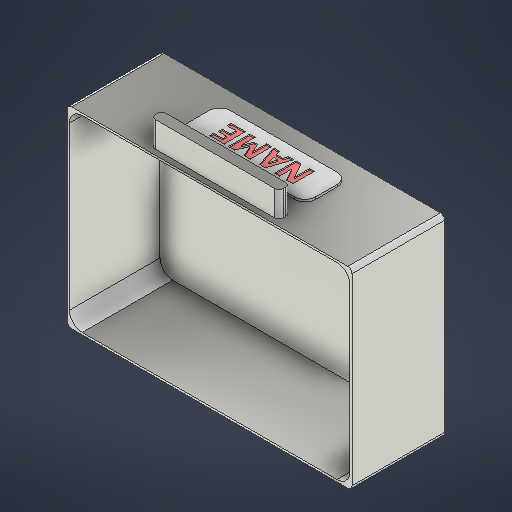
# Autodesk Inventor part: shelf1x2
Saved by Autodesk Inventor 2027 (Build 310192060, 192F)
## iProperties
Created: 2026-06-08
Part Number: shelf1x2
Material: Ogólny
Document SubType Name: Modeling
Designer: User
Density: 1 g/cm^3
Appearance: Domyślna
Author: User
Autodesk Inventor part; units mm, degrees
ref_plane "YZ Plane" through (0, 0, 0) normal (1, 0, 0) x (0, 1, 0)
ref_plane "XZ Plane" through (0, 0, 0) normal (0, 1, 0) x (-1, 0, 0)
ref_plane "XY Plane" through (0, 0, 0) normal (0, 0, 1) x (1, 0, 0)
sketch "Szkic1" plane through (0, 0, 0) normal (0, 1, 0) x (-1, 0, 0)
  line L0 (-66.7, -21.7) -> (66.7, -21.7)
  line L1 (66.7, -21.7) -> (66.7, 21.7)
  line L2 (66.7, 21.7) -> (-66.7, 21.7)
  line L3 (-66.7, 21.7) -> (-66.7, -21.7)
  line L4 (-66.7, -21.7) -> (66.7, 21.7) construction
  line L5 (66.7, -21.7) -> (-66.7, 21.7) construction
  point P0 (0, 0)
  dimension "d0" = 133.4
  dimension "d1" = 43.4
  constraints: 12 end point, 2 midpoint, 2 parallel, 1 horizontal, 1 perpendicular
  measures "d0" distance of L2.end L1.end
  measures "d1" distance of L1.end L0.end
extrude "Wyciągnięcie proste1" add sketch "Szkic1" along normal blind 90
shell "Skorupa1" thickness 1 removed faces 1 at (-22.2333, 30, 21.7)
sketch "Szkic2" plane through (0, 90, 0) normal (0, 1, 0) x (1, 0, 0)
  line L0 (-66.7, -21.7) -> (66.7, -21.7) projected
  line L1 (0, -21.7) -> (0, -16.7)
  line L2 (30, -19.2) -> (-30, -19.2)
  line L3 (-30, -19.2) -> (-30, -14.2)
  line L4 (-30, -14.2) -> (30, -14.2)
  line L5 (30, -14.2) -> (30, -19.2)
  line L6 (30, -19.2) -> (-30, -14.2) construction
  line L7 (-30, -19.2) -> (30, -14.2) construction
  point P0 (0, 0)
  dimension "d5" = 5
  dimension "d6" = 60
  dimension "d7" = 5
  constraints: 14 end point, 3 midpoint, 2 parallel, 1 horizontal, 1 perpendicular, 1 vertical
  measures "d5" distance of L1.start L1.end
  measures "d6" distance of L2.start L2.end
  measures "d7" distance of L2.end L3.end
extrude "Wyciągnięcie proste2" add sketch "Szkic2" along normal blind 12
sketch "Szkic3" plane through (0, 90, 0) normal (0, 1, 0) x (1, 0, 0)
  line L0 (0, 0) -> (0, 3)
  line L1 (30, 13) -> (-30, 13)
  line L2 (-30, 13) -> (-30, -7)
  line L3 (-30, -7) -> (30, -7)
  line L4 (30, -7) -> (30, 13)
  line L5 (30, 13) -> (-30, -7) construction
  line L6 (-30, 13) -> (30, -7) construction
  dimension "d10" = 3
  dimension "d11" = 60
  dimension "d12" = 20
  constraints: 14 end point, 2 midpoint, 2 parallel, 1 horizontal, 1 perpendicular, 1 vertical
  measures "d10" distance of L0.start L0.end
  measures "d11" distance of L3.end L2.end
  measures "d12" distance of L2.end L1.end
extrude "Wyciągnięcie proste3" add sketch "Szkic3" along normal blind 1
sketch "Szkic4" plane through (0, 91, 0) normal (0, 1, 0) x (1, 0, 0)
  line L0 (30, -7) -> (-30, -7) construction
  line L1 (-30, -7) -> (-30, 13) construction
  line L2 (-30, 13) -> (30, 13) construction
  line L3 (30, 13) -> (30, -7) construction
  line L4 (-30, -7) -> (30, -7) projected
  line L5 (-30, 13) -> (-30, -7) projected
  line L6 (30, -7) -> (-30, -7)
  line L7 (-30, -7) -> (-30, 13)
  line L8 (-30, 13) -> (30, 13)
  line L9 (30, 13) -> (30, -7)
  line L10 (10.778, 8) -> (13.1929, 8)
  line L11 (13.1929, 8) -> (17.0502, 1.0308)
  line L12 (17.0502, 1.0308) -> (17.0502, 8)
  line L13 (17.0502, 8) -> (19.3436, 8)
  line L14 (19.3436, 8) -> (19.3436, -2)
  line L15 (19.3436, -2) -> (16.2642, -2)
  line L16 (16.2642, -2) -> (13.0713, 3.7293)
  line L17 (13.0713, 3.7293) -> (13.0713, -2)
  line L18 (13.0713, -2) -> (10.778, -2)
  line L19 (10.778, -2) -> (10.778, 8)
  line L20 (9.8217, 8) -> (6.4425, -2)
  line L21 (6.4425, -2) -> (3.7034, -2)
  line L22 (3.7034, -2) -> (0.3241, 8)
  line L23 (0.3241, 8) -> (2.9092, 8)
  line L24 (2.9092, 8) -> (3.5332, 5.9579)
  line L25 (3.5332, 5.9579) -> (6.6775, 5.9579)
  line L26 (6.6775, 5.9579) -> (7.3096, 8)
  line L27 (7.3096, 8) -> (9.8217, 8)
  line L28 (4.0843, 4.1426) -> (5.1053, 0.8363)
  line L29 (5.1053, 0.8363) -> (6.1345, 4.1426)
  line L30 (6.1345, 4.1426) -> (4.0843, 4.1426)
  line L31 (-10.8833, 8) -> (-8.3874, 8)
  line L32 (-8.3874, 8) -> (-8.3874, 1.3712)
  line L33 (-8.3874, 1.3712) -> (-6.5721, 5.6499)
  line L34 (-6.5721, 5.6499) -> (-4.8541, 5.6499)
  line L35 (-4.8541, 5.6499) -> (-3.0389, 1.3712)
  line L36 (-3.0389, 1.3712) -> (-3.0389, 8)
  line L37 (-3.0389, 8) -> (-0.6726, 8)
  line L38 (-0.6726, 8) -> (-0.6726, -2)
  line L39 (-0.6726, -2) -> (-3.5656, -2)
  line L40 (-3.5656, -2) -> (-5.7861, 2.9352)
  line L41 (-5.7861, 2.9352) -> (-7.9903, -2)
  line L42 (-7.9903, -2) -> (-10.8833, -2)
  line L43 (-10.8833, -2) -> (-10.8833, 8)
  line L44 (-12.9579, 8) -> (-12.9579, -2)
  line L45 (-12.9579, -2) -> (-19.7164, -2)
  line L46 (-19.7164, -2) -> (-19.7164, -0.0956)
  line L47 (-19.7164, -0.0956) -> (-15.4538, -0.0956)
  line L48 (-15.4538, -0.0956) -> (-15.4538, 1.6629)
  line L49 (-15.4538, 1.6629) -> (-19.3841, 1.6629)
  line L50 (-19.3841, 1.6629) -> (-19.3841, 3.5673)
  line L51 (-19.3841, 3.5673) -> (-15.4538, 3.5673)
  line L52 (-15.4538, 3.5673) -> (-15.4538, 6.0956)
  line L53 (-15.4538, 6.0956) -> (-19.7164, 6.0956)
  line L54 (-19.7164, 6.0956) -> (-19.7164, 8)
  line L55 (-19.7164, 8) -> (-12.9579, 8)
  point P0 (0, 0)
  dimension "d0" = 133.4
  dimension "d1" = 43.4
  constraints: 8 end point, 2 coincident, 2 parallel, 1 horizontal, 1 perpendicular, 2 other
extrude "Wyciągnięcie proste4" cut sketch "Szkic4" against normal blind 0.6 contours L10 L11 L12 L13 L14 L15 L16 L17 L18 L19 | L20 L21 L22 L23 L24 L25 L26 L27 | L31 L32 L33 L34 L35 L36 L37 L38 L39 L40 L41 L42 L43 | L44 L45 L46 L47 L48 L49 L50 L51 L52 L53 L54 L55
fillet "Zaokrąglenie1" radius 5 4 edges at (-30, 90.5, 7) (-30, 90.5, -13) (30, 90.5, 7) (30, 90.5, -13)
fillet "Zaokrąglenie2" radius 6 4 edges at (65.7, 1, 0.5) (-65.7, 1, 0.5) (65.7, 89, 0.5) (-65.7, 89, 0.5)
fillet "Zaokrąglenie3" radius 2 4 edges at (66.7, 90, 0) (-66.7, 90, 0) (-66.7, 0, 0) (66.7, 0, 0)
fillet "Zaokrąglenie4" radius 2 4 edges at (-30, 96, 14.2) (-30, 96, 19.2) (30, 96, 14.2) (30, 96, 19.2)
